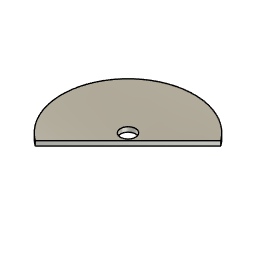
Washer half (Autodesk Fusion 360 design; units mm, degrees)
Autodesk Fusion 360 part; units mm, degrees
note: some values were not read from the file. Set by a fixed rule: which sketch regions a step uses.
sketch "スケッチ1" plane through (0, 0, 0) normal (0, 0, 1) x (1, 0, 0)
  circle A0 centre (0, 0) radius 14
  circle A1 centre (0, 0) radius 1.6
  line L0 (0, 0) -> (1.4142, -1.4142)
  line L1 (1.4142, -1.4142) -> (11.2122, 8.3837)
  line L2 (1.4142, -1.4142) -> (-8.3837, -11.2122)
  dimension "d1" = 28
  dimension "d2" = 3.2
  dimension "d3" = 2
  constraint coincident A0.centre A1.centre
  constraint concentric A0 A1
  constraint coincident A0 L1.end
  constraint perpendicular L0 L1
  constraint coincident A0 L2.end
  constraint perpendicular L0 L2
  measures "d1" diameter of A0
  measures "d2" diameter of A1
  measures "d3" distance of A0.centre L0.end
extrude "押し出し1" add sketch "スケッチ1" along normal blind 1 contours A0 L1 L2 picked at (-6.457, -7.4261)
